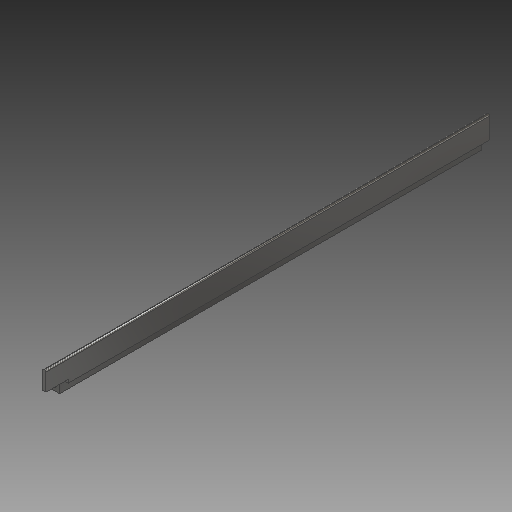
# Autodesk Inventor part: gancho
Saved by Autodesk Inventor 2019 (Build 230136000, 136)
## iProperties
Created: 2019-03-24
Part Number: gancho
Material: Generic
Document SubType Name: Modeling
Designer: felix
Density: 1 g/cm^3
Appearance: Default
Mass: 195.581 g
Surface Area: 911.764 cm^2
Volume: 195.581 cm^3
Author: felix
Autodesk Inventor part; units mm, degrees
sketch "Sketch1" plane through (0, 0, 0) normal (0, 0, 1) x (1, 0, 0)
  line L0 (0, 0) -> (-20.5, 0)
  line L1 (-20.5, 0) -> (-20.5, 48)
  line L2 (11.5, 18) -> (0, 18)
  line L3 (0, 18) -> (0, 0)
  line L4 (-20.5, 48) -> (11.5, 48)
  line L5 (11.5, 48) -> (11.5, 18)
  line L6 (-20.5, 0) -> (0, 0)
  line L7 (0, 0) -> (0, 3.5)
  line L8 (-20.5, 3.5) -> (-20.5, 0)
  line L9 (0, 18) -> (11.5, 18)
  line L10 (11.5, 18) -> (11.5, 21.0352)
  line L11 (-20.5, 0) -> (0, 0)
  line L12 (0, 0) -> (0, 4.5)
  line L13 (-20.5, 4.5) -> (-20.5, 0)
  line L14 (-4.5, 22.5) -> (-4.5, 4.5)
  line L15 (-4.5, 4.5) -> (-20.5, 4.5)
  line L16 (-4.5, 22.5) -> (7, 22.5)
  line L17 (7, 22.5) -> (7, 48)
  point P0 (-2.8995, 48)
  dimension "d0" = 20.5
  dimension "d1" = 48
  dimension "d9" = 30
  dimension "d10" = 32
  dimension "d11" = 11.5
  dimension "d16" = 16
  dimension "d23" = 4.5
  dimension "d24" = 4.5
  dimension "d25" = 4.5
  constraints: 36 end point, 6 perpendicular, 5 horizontal, 5 point on line, 4 parallel, 2 vertical
  measures "d0" distance of L0.start L0.end
  measures "d1" distance of L0.end L1.end
  measures "d9" distance of L4.end L2.start
  measures "d10" distance of L1.end L4.end
  measures "d11" distance of L2.start L2.end
  measures "d16" distance of L14.end L13.start
  measures "d23" distance between parallel lines of L0 L15
  measures "d24" distance between parallel lines of L9 L16
  measures "d25" distance between parallel lines of L5 L17
extrude "Extrusion2" add sketch "Sketch1" along normal blind 600 contours L0 L1 L15 L14 L16 L17 L4 L5 L2 L3
ref_plane "Work Plane4" through (-4.5, 7.5, 0) normal (-1, 0, 0) x (0, 0, 1)
ref_plane "Work Plane3" through (-4.5, 7.5, 0) normal (-1, 0, 0) x (0, 0, 1)
ref_plane "Work Plane2" through (-4.5, 7.5, 0) normal (-1, 0, 0) x (0, 0, 1)
ref_plane "Work Plane1" through (-4.5, 7.5, 0) normal (-1, 0, 0) x (0, 0, 1)
sketch "Sketch7" plane through (-20.5, 0, 0) normal (-1, 0, 0) x (0, 0, 1)
  line L0 (600, 22.5) -> (600, 4.5) projected
  line L1 (0, 0) -> (600, 0) projected
  line L2 (660, 22.5) -> (0, 22.5) projected
  line L3 (600, 0) -> (570, 0)
  line L4 (570, 0) -> (570, 22.5)
  line L5 (570, 22.5) -> (600, 22.5)
  line L6 (600, 22.5) -> (600, 0)
  point P0 (660, 19.5)
  point P1 (660, 7.5)
  dimension "d71" = 30
  constraints: 8 end point, 2 parallel, 1 horizontal, 1 perpendicular, 1 point on line, 1 other
  measures "d71" distance of L4.end L5.end
extrude "Extrusion4" cut sketch "Sketch7" along normal mid plane 1000
fillet "Fillet4" radius 2 5 edges at (-20.5, 4.5, 285) (-4.5, 22.5, 285) (7, 48, 300) (11.5, 48, 300) (-4.5, 4.5, 285)
body "Solid2"
